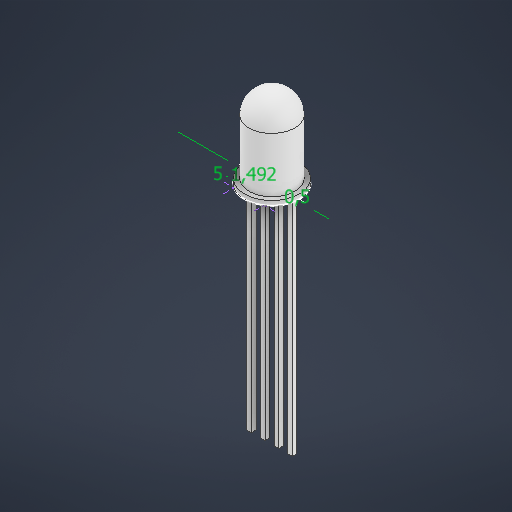
# Autodesk Inventor part: ESP32_C3_SM
Saved by Autodesk Inventor 2026.2 (Build 302298010, 298A)
## iProperties
Created: 2026-05-20
Part Number: ESP32_C3_SM
Material: ABS Plastic
Document SubType Name: Modeling
Designer: anton
Density: 1.06 g/cm^3
Appearance: Smooth - White
Author: anton
Autodesk Inventor part; units mm, degrees
ref_plane "YZ Plane" through (0, 0, 0) normal (1, 0, 0) x (0, 1, 0)
ref_plane "XZ Plane" through (0, 0, 0) normal (0, 1, 0) x (-1, 0, 0)
ref_plane "XY Plane" through (0, 0, 0) normal (0, 0, 1) x (1, 0, 0)
sketch "Sketch1" plane through (0, 0, 0) normal (0, 1, 0) x (-1, 0, 0)
  circle A0 centre (0, 0) radius 2.5
  circle A1 centre (0, 0) radius 3
  line L0 (1.9875, 0.25) -> (2.4875, 0.25)
  line L1 (2.4875, 0.25) -> (2.4875, -0.25)
  line L2 (2.4875, -0.25) -> (1.9875, -0.25)
  line L3 (1.9875, -0.25) -> (1.9875, 0.25)
  line L4 (1.9875, 0.25) -> (2.4875, -0.25) construction
  line L5 (2.4875, 0.25) -> (1.9875, -0.25) construction
  line L6 (2.5, 0) -> (-2.5, 0)
  line L7 (0.9958, 0.25) -> (0.9958, -0.25)
  line L8 (0.4958, 0.25) -> (0.9958, 0.25)
  line L9 (0.4958, -0.25) -> (0.4958, 0.25)
  line L10 (0.9958, -0.25) -> (0.4958, -0.25)
  line L11 (0.9958, 0.25) -> (0.4958, -0.25) construction
  line L12 (0.4958, 0.25) -> (0.9958, -0.25) construction
  line L13 (-0.4958, 0.25) -> (-0.4958, -0.25)
  line L14 (-0.9958, 0.25) -> (-0.4958, 0.25)
  line L15 (-0.9958, -0.25) -> (-0.9958, 0.25)
  line L16 (-0.4958, -0.25) -> (-0.9958, -0.25)
  line L17 (-0.4958, 0.25) -> (-0.9958, -0.25) construction
  line L18 (-0.9958, 0.25) -> (-0.4958, -0.25) construction
  line L19 (-1.9875, 0.25) -> (-1.9875, -0.25)
  line L20 (-2.4875, 0.25) -> (-1.9875, 0.25)
  line L21 (-2.4875, -0.25) -> (-2.4875, 0.25)
  line L22 (-1.9875, -0.25) -> (-2.4875, -0.25)
  line L23 (-1.9875, 0.25) -> (-2.4875, -0.25) construction
  line L24 (-2.4875, 0.25) -> (-1.9875, -0.25) construction
  point P0 (1.6583, 2.5)
  point P1 (-1.6583, 2.5)
  point P2 (2.2375, 0)
  point P3 (0.7458, 0)
  point P4 (-0.7458, 0)
  point P5 (-2.2375, 0)
  dimension "d11" = 5
  dimension "d12" = 0.5
  dimension "d22" = 1.4916
  constraints: 50 end point, 5 point on circle, 4 horizontal, 2 centre point, 2 midpoint, 2 parallel, 2 perpendicular, 1 coincident, 1 collinear, 1 point on line, 32 other
  measures "d11" diameter of A0
  measures "d12" radial gap between concentric circles of A0 A1
  measures "d22" distance of L0.end L7.start
extrude "Extrusion3" add sketch "Sketch1" along normal blind 9 contours L6 L1 A0 | A0 L1 L6 | L0 L3 L6 L7 L8 L9 L13 L14 L15 L19 L20 A0 | L1 L6 L3 L0 | L2 L3 L6 L1 | A0 L22 L19 L6 L15 L16 L13 L9 L10 L7 L3 L2 | L21 L6 A0 | L20 L19 L6 L21 | A0 L6 L21 | L21 L6 L19 L22 | L7 L10 L9 L6 | L6 L9 L8 L7 | L15 L14 L13 L6 | L6 L13 L16 L15
extrude "Extrusion4" add sketch "Sketch1" along normal blind 0.5
fillet "Fillet2" radius 2.5 1 edges at (2.5, 9, 0)
extrude "Extrusion5" add sketch "Sketch1" against normal blind 24.5 contours L1 L6 L3 L0 | L2 L3 L6 L1 | L20 L19 L6 L21 | L21 L6 L19 L22 | L7 L10 L9 L6 | L6 L9 L8 L7 | L15 L14 L13 L6 | L6 L13 L16 L15
body "Solid3"
